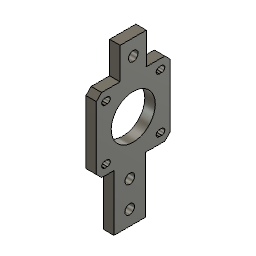
motor_mount_ed (Autodesk Fusion 360 design; units mm, degrees)
Autodesk Fusion 360 part; units mm, degrees
sketch "Sketch1" plane through (0, 0, 0) normal (1, 0, 0) x (0, 0, -1)
  line L0 (-21, 21) -> (21, 21)
  line L1 (21, 21) -> (21, -21)
  line L2 (21, -21) -> (-21, -21)
  line L3 (-21, -21) -> (-21, 21)
  line L4 (-11, -21) -> (7, -21)
  line L5 (7, -53) -> (-11, -53)
  line L6 (-11, -53) -> (-11, -21)
  line L7 (-21, 0) -> (21, 0) construction
  circle A0 centre (0, 0) radius 12.5
  circle A1 centre (-2, -29.5) radius 2.75
  circle A2 centre (-2, -44.5) radius 2.75
  line L8 (-2, -44.5) -> (-2, -29.5) construction
  line L9 (-16.25, 17.2) -> (-14.75, 17.2)
  arc A3 (-14.75, 13.8) -> (-14.75, 17.2) centre (-14.75, 15.5) ccw
  line L10 (-14.75, 13.8) -> (-16.25, 13.8)
  arc A4 (-16.25, 17.2) -> (-16.25, 13.8) centre (-16.25, 15.5) ccw
  line L11 (-14.75, 15.5) -> (-16.25, 15.5) construction
  line L12 (0, 20) -> (0, 2.5)
  line L13 (14.75, 13.8) -> (16.25, 13.8)
  arc A5 (16.25, 13.8) -> (16.25, 17.2) centre (16.25, 15.5) ccw
  line L14 (16.25, 17.2) -> (14.75, 17.2)
  arc A6 (14.75, 17.2) -> (14.75, 13.8) centre (14.75, 15.5) ccw
  arc A7 (-14.75, -17.2) -> (-14.75, -13.8) centre (-14.75, -15.5) ccw
  line L15 (-14.75, -13.8) -> (-16.25, -13.8)
  arc A8 (-16.25, -13.8) -> (-16.25, -17.2) centre (-16.25, -15.5) ccw
  line L16 (-16.25, -17.2) -> (-14.75, -17.2)
  arc A9 (14.75, -13.8) -> (14.75, -17.2) centre (14.75, -15.5) ccw
  line L17 (16.25, -17.2) -> (14.75, -17.2)
  arc A10 (16.25, -17.2) -> (16.25, -13.8) centre (16.25, -15.5) ccw
  line L18 (14.75, -13.8) -> (16.25, -13.8)
  line L19 (7, -53) -> (7, -21)
  point P0 (-2, -53)
  point P1 (-2, -37)
  point P2 (-15.5, 15.5)
  dimension "d1" = 42
  dimension "d4" = 42
  dimension "d8" = 25
  dimension "d9" = 5.5
  dimension "d12" = 5.5
  dimension "d13" = 15
  dimension "d28" = 1.5
  dimension "d29" = 15.5
  dimension "d30" = 15.5
  dimension "d31" = 1.7
  dimension "d32" = 32
  dimension "d33" = 18
  dimension "d34" = 16
  dimension "d35" = 2
  constraint horizontal L0
  constraint vertical L1
  constraint horizontal L2
  constraint vertical L3
  constraint horizontal L4
  constraint horizontal L5
  constraint vertical L6
  constraint midpoint L3 L7.start
  constraint midpoint L1 L7.end
  constraint midpoint L7 A0.centre
  constraint coincident A0.centre origin
  constraint midpoint L5 P0
  constraint coincident A2.centre L8.start
  constraint coincident A1.centre L8.end
  constraint midpoint L8 P1
  constraint tangent L9 A3
  constraint tangent L10 A4
  constraint horizontal L9
  constraint tangent A3 L10
  constraint horizontal L10
  constraint coincident L9.start A4.start
  constraint tangent L9 A4
  constraint coincident A3.centre L11.start
  constraint coincident A4.centre L11.end
  constraint midpoint L11 P2
  constraint symmetric L9.start L12 A5.end
  constraint symmetric L9.end L12 L14.end
  constraint symmetric A3.start L12 L13.start
  constraint symmetric A3 L12 A6
  constraint symmetric L10.end L12 L13.end
  constraint symmetric A4 L12 A5
  constraint symmetric L7 L9.start A8.end
  constraint symmetric L7 L9.end A7.start
  constraint symmetric L7 A3.start A7.end
  constraint symmetric L7 A3 A7
  constraint symmetric L7 L10.end L15.end
  constraint symmetric L7 A4 A8
  constraint symmetric L7 L13.start A9.start
  constraint symmetric L7 L13.end A10.end
  constraint symmetric L7 A5.end L17.start
  constraint symmetric L7 A5 A10
  constraint symmetric L7 L14.end A9.end
  constraint symmetric L7 A6 A9
  constraint vertical L19
  constraint coincident L1.end L2.start
  constraint coincident L2 L4.end
  constraint vertical L8
  constraint vertical P0 P1
  measures "d1" distance of L0.start L0.end
  measures "d4" distance of L0.end L1.end
  measures "d8" diameter of A0
  measures "d9" diameter of A1
  measures "d12" diameter of A2
  measures "d13" distance of A1.centre A2.centre
  measures "d28" distance of A3.centre A4.centre
  measures "d29" vertical distance of A0.centre P2
  measures "d30" horizontal distance of A0.centre P2
  measures "d31" radius of A3
  measures "d32" distance of L5.start L4.end
  measures "d33" distance of L5.start L5.end
  measures "d34" vertical distance of L1.end P1
  measures "d35" horizontal distance of A0.centre P1
extrude "Extrude1" add sketch "Sketch1" along normal blind 6
sketch "Sketch4" plane through (0, 0, 0) normal (-1, 0, 0) x (0, 0, 1)
  circle A0 centre (0, 0) radius 12.5
  line L0 (21, -21) -> (21, 21)
  line L1 (21, 21) -> (-21, 21)
  line L2 (-7.5, 21) -> (7.5, 21)
  line L3 (7.5, 21) -> (7.5, 39)
  line L4 (7.5, 39) -> (-7.5, 39)
  line L5 (-7.5, 39) -> (-7.5, 21)
  line L6 (-21, 21) -> (-21, -21)
  line L7 (-21, -21) -> (-7, -21)
  circle A1 centre (2, -44.5) radius 2.75
  circle A2 centre (2, -29.5) radius 2.75
  line L8 (-7, -53) -> (11, -53)
  line L9 (11, -53) -> (11, -21)
  line L10 (11, -21) -> (21, -21)
  line L11 (-7, -21) -> (-7, -53)
  arc A3 (-14.75, 13.8) -> (-14.75, 17.2) centre (-14.75, 15.5) ccw
  line L12 (-14.75, 13.8) -> (-16.25, 13.8)
  arc A4 (-16.25, 17.2) -> (-16.25, 13.8) centre (-16.25, 15.5) ccw
  line L13 (-16.25, 17.2) -> (-14.75, 17.2)
  line L14 (16.25, -17.2) -> (14.75, -17.2)
  arc A5 (14.75, -13.8) -> (14.75, -17.2) centre (14.75, -15.5) ccw
  line L15 (14.75, -13.8) -> (16.25, -13.8)
  arc A6 (16.25, -17.2) -> (16.25, -13.8) centre (16.25, -15.5) ccw
  arc A7 (-16.25, -13.8) -> (-16.25, -17.2) centre (-16.25, -15.5) ccw
  line L16 (-16.25, -13.8) -> (-14.75, -13.8)
  arc A8 (-14.75, -17.2) -> (-14.75, -13.8) centre (-14.75, -15.5) ccw
  line L17 (-14.75, -17.2) -> (-16.25, -17.2)
  arc A9 (14.75, 17.2) -> (14.75, 13.8) centre (14.75, 15.5) ccw
  line L18 (14.75, 17.2) -> (16.25, 17.2)
  arc A10 (16.25, 13.8) -> (16.25, 17.2) centre (16.25, 15.5) ccw
  line L19 (16.25, 13.8) -> (14.75, 13.8)
  point P0 (0, 21)
  dimension "d18" = 18
  dimension "d19" = 15
  constraint horizontal L2
  constraint vertical L3
  constraint horizontal L4
  constraint vertical L5
  constraint coincident L1 L2.start
  constraint midpoint L2 P0
  constraint vertical A0.centre P0
  measures "d18" distance of L2.start L4.end
  measures "d19" distance of L3.end L4.end
extrude "Extrude2" add sketch "Sketch4" against normal up to surface (6 mm away) contours L1 L2 L3 L4 L5
sketch "Sketch5" plane through (0, 0, 0) normal (-1, 0, 0) x (0, 0, 1)
  circle A0 centre (0, 0) radius 12.5
  line L0 (21, -21) -> (21, 21)
  line L1 (21, 21) -> (7.5, 21)
  line L2 (7.5, 21) -> (7.5, 39)
  line L3 (7.5, 39) -> (-7.5, 39)
  line L4 (-7.5, 39) -> (-7.5, 21)
  line L5 (-7.5, 21) -> (-21, 21)
  circle A1 centre (0, 30) radius 2.75
  line L6 (-21, 21) -> (-21, -21)
  line L7 (-21, -21) -> (-7, -21)
  circle A2 centre (2, -44.5) radius 2.75
  circle A3 centre (2, -29.5) radius 2.75
  line L8 (-7, -53) -> (11, -53)
  line L9 (11, -53) -> (11, -21)
  line L10 (11, -21) -> (21, -21)
  line L11 (-7, -21) -> (-7, -53)
  arc A4 (-14.75, 13.8) -> (-14.75, 17.2) centre (-14.75, 15.5) ccw
  line L12 (-14.75, 13.8) -> (-16.25, 13.8)
  arc A5 (-16.25, 17.2) -> (-16.25, 13.8) centre (-16.25, 15.5) ccw
  line L13 (-16.25, 17.2) -> (-14.75, 17.2)
  line L14 (16.25, -17.2) -> (14.75, -17.2)
  arc A6 (14.75, -13.8) -> (14.75, -17.2) centre (14.75, -15.5) ccw
  line L15 (14.75, -13.8) -> (16.25, -13.8)
  arc A7 (16.25, -17.2) -> (16.25, -13.8) centre (16.25, -15.5) ccw
  arc A8 (-16.25, -13.8) -> (-16.25, -17.2) centre (-16.25, -15.5) ccw
  line L16 (-16.25, -13.8) -> (-14.75, -13.8)
  arc A9 (-14.75, -17.2) -> (-14.75, -13.8) centre (-14.75, -15.5) ccw
  line L17 (-14.75, -17.2) -> (-16.25, -17.2)
  arc A10 (14.75, 17.2) -> (14.75, 13.8) centre (14.75, 15.5) ccw
  line L18 (14.75, 17.2) -> (16.25, 17.2)
  arc A11 (16.25, 13.8) -> (16.25, 17.2) centre (16.25, 15.5) ccw
  line L19 (16.25, 13.8) -> (14.75, 13.8)
  dimension "d22" = 30
  dimension "d23" = 5.5
  constraint vertical A0.centre A1.centre
  measures "d22" vertical distance of A0.centre A1.centre
  measures "d23" diameter of A1
extrude "Extrude3" cut sketch "Sketch5" against normal blind 30 contours A1
chamfer "Chamfer1" distance 3 angle 45 4 edges at (3, 21, 21) (3, -21, 21) (3, -21, -21) (3, 21, -21)
sketch "Sketch6" plane through (6, 0, 0) normal (1, 0, 0) x (0, 0, -1)
  line L0 (18, 21) -> (7.5, 21)
  line L1 (7.5, 21) -> (7.5, 39)
  line L2 (7.5, 39) -> (-7.5, 39)
  line L3 (-7.5, 39) -> (-7.5, 21)
  line L4 (-7.5, 21) -> (-18, 21)
  line L5 (-18, 21) -> (-21, 18)
  line L6 (-21, 18) -> (-21, -18)
  circle A0 centre (0, 0) radius 12.5
  circle A1 centre (0, 30) radius 2.75
  line L7 (7, -21) -> (18, -21)
  line L8 (21, -18) -> (21, 18)
  circle A2 centre (-2, -44.5) radius 2.75
  circle A3 centre (-2, -29.5) radius 2.75
  line L9 (-21, -18) -> (-18, -21)
  line L10 (-18, -21) -> (-11, -21)
  line L11 (-11, -21) -> (-11, -53)
  line L12 (-11, -53) -> (7, -53)
  line L13 (7, -53) -> (7, -21)
  line L14 (21, 18) -> (18, 21)
  line L15 (18, -21) -> (21, -18)
  arc A4 (14.75, 17.2) -> (14.75, 13.8) centre (14.75, 15.5) ccw
  line L16 (14.75, 17.2) -> (16.25, 17.2)
  arc A5 (16.25, 13.8) -> (16.25, 17.2) centre (16.25, 15.5) ccw
  line L17 (16.25, 13.8) -> (14.75, 13.8)
  line L18 (-14.75, -17.2) -> (-16.25, -17.2)
  arc A6 (-16.25, -13.8) -> (-16.25, -17.2) centre (-16.25, -15.5) ccw
  line L19 (-16.25, -13.8) -> (-14.75, -13.8)
  arc A7 (-14.75, -17.2) -> (-14.75, -13.8) centre (-14.75, -15.5) ccw
  arc A8 (16.25, -17.2) -> (16.25, -13.8) centre (16.25, -15.5) ccw
  line L20 (16.25, -17.2) -> (14.75, -17.2)
  arc A9 (14.75, -13.8) -> (14.75, -17.2) centre (14.75, -15.5) ccw
  line L21 (14.75, -13.8) -> (16.25, -13.8)
  arc A10 (-14.75, 13.8) -> (-14.75, 17.2) centre (-14.75, 15.5) ccw
  line L22 (-14.75, 13.8) -> (-16.25, 13.8)
  arc A11 (-16.25, 17.2) -> (-16.25, 13.8) centre (-16.25, 15.5) ccw
  line L23 (-16.25, 17.2) -> (-14.75, 17.2)
equation "d31 = 3.4 mm / 2"
